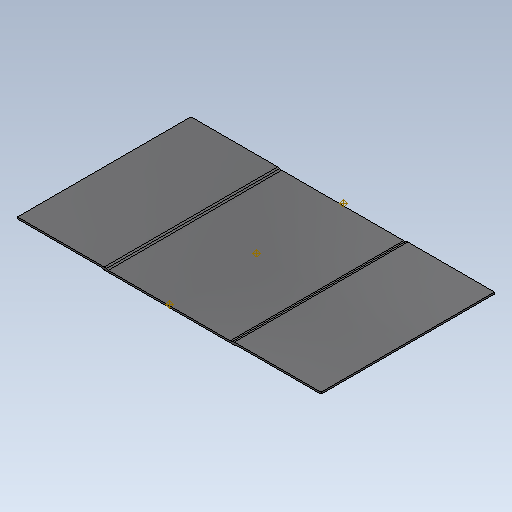
# Autodesk Inventor part: Ribbon Tape
Saved by Autodesk Inventor 2020.1 (Build 241239000, 239)
## iProperties
Created: 2009-10-16
Part Number: Ribbon Tape
Document SubType Name: Modeling
Designer: Thom Tremblay
Density: 1 g/cm^3
Material: Generic
Appearance: Smooth - Medium Gray
Author: Thom Tremblay
Autodesk Inventor part; units mm, degrees
ref_plane "YZ Plane" through (0, 0, 0) normal (1, 0, 0) x (0, 1, 0)
ref_plane "XZ Plane" through (0, 0, 0) normal (0, 1, 0) x (-1, 0, 0)
ref_plane "XY Plane" through (0, 0, 0) normal (0, 0, 1) x (1, 0, 0)
sketch "Sketch1" plane through (0, 0, 0) normal (0, 0, 1) x (1, 0, 0)
  line L0 (-22.225, 0) -> (-9.525, 0)
  line L1 (-9.525, 0) -> (-9.525, -0.254)
  line L2 (-9.525, -0.254) -> (-22.225, -0.254)
  line L3 (-22.225, -0.254) -> (-22.225, 0)
  line L4 (-9.525, -0.127) -> (9.525, -0.127)
  line L5 (9.525, -0.127) -> (9.525, -0.381)
  line L6 (9.525, -0.381) -> (-9.525, -0.381)
  line L7 (-9.525, -0.381) -> (-9.525, -0.127)
  line L8 (9.525, -0.254) -> (22.225, -0.254)
  line L9 (22.225, -0.254) -> (22.225, 0)
  line L10 (22.225, 0) -> (9.525, 0)
  line L11 (9.525, 0) -> (9.525, -0.254)
  line L12 (0, -0.127) -> (0, 0) construction
  arc A0 (-9.8215, -0.3175) -> (-9.525, -0.381) centre (-9.525, 0.343) ccw
  arc A1 (-9.8215, -0.3175) -> (-10.118, -0.254) centre (-10.118, -0.978) ccw
  arc A2 (-9.2285, -0.0635) -> (-9.525, 0) centre (-9.525, -0.724) ccw
  arc A3 (-9.2285, -0.0635) -> (-8.932, -0.127) centre (-8.932, 0.597) ccw
  arc A4 (9.525, -0.381) -> (9.8215, -0.3175) centre (9.525, 0.343) ccw
  arc A5 (10.118, -0.254) -> (9.8215, -0.3175) centre (10.118, -0.978) ccw
  arc A6 (9.525, 0) -> (9.2285, -0.0635) centre (9.525, -0.724) ccw
  arc A7 (8.932, -0.127) -> (9.2285, -0.0635) centre (8.932, 0.597) ccw
  dimension "d0" = 12.7
  dimension "d1" = 19.05
  dimension "d2" = 0.254
  constraints: 26 end point, 16 point on circle, 12 tangent, 8 centre point, 7 equal radius, 7 parallel, 5 point on line, 3 equal length, 3 horizontal, 3 midpoint, 3 perpendicular, 1 coincident
  measures "d0" distance of L9.end L10.end
  measures "d1" distance of L5.end L6.end
  measures "d2" distance of L8.end L9.end
extrude "Extrusion1" add sketch "Sketch1" along normal mid plane 25.4
sketch "Sketch2" plane through (0, 0, -12.7) normal (0, 0, -1) x (-1, 0, 0)
  point P0 (0, 0)
sketch "Sketch3" plane through (0, 0, 12.7) normal (0, 0, 1) x (1, 0, 0)
  point P0 (0, 0)
body "Solid1"
